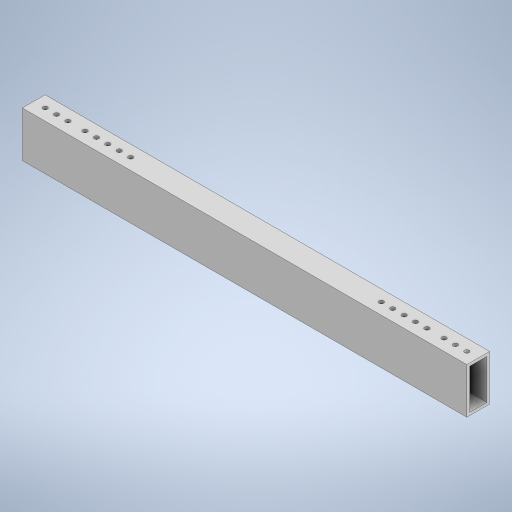
# Autodesk Inventor part: (a)swerveassembly
Saved by Autodesk Inventor 2024 (Build 280153000, 153)
## iProperties
Created: 2023-09-27
Part Number: (a)swerveassembly
Material: Generic
Document SubType Name: Modeling
Designer: s137416
Density: 1 g/cm^3
Appearance: Default
Author: s137416
Autodesk Inventor part; units mm, degrees
ref_plane "YZ Plane" through (0, 0, 0) normal (1, 0, 0) x (0, 1, 0)
ref_plane "XZ Plane" through (0, 0, 0) normal (0, 1, 0) x (-1, 0, 0)
ref_plane "XY Plane" through (0, 0, 0) normal (0, 0, 1) x (1, 0, 0)
sketch "Sketch1" plane through (0, 0, 0) normal (0, 0, 1) x (1, 0, 0)
  line L0 (-7.3593, 50.2532) -> (487.9407, 50.2532)
  line L1 (487.9407, 50.2532) -> (487.9407, -0.5468)
  line L2 (487.9407, -0.5468) -> (-7.3593, -0.5468)
  line L3 (-7.3593, -0.5468) -> (-7.3593, 50.2532)
  point P0 (0, 0)
  dimension "d0" = 495.3
  dimension "d1" = 50.8
  constraints: 8 end point, 2 parallel, 1 horizontal, 1 perpendicular
  measures "d0" distance of L1.end L2.end
  measures "d1" distance of L2.end L0.start
extrude "Extrusion1" add sketch "Sketch1" along normal blind 25.4
sketch "Sketch2" plane through (-7.3593, 50.2532, 0) normal (0, 1, 0) x (1, 0, 0)
  circle A0 centre (57.15, -12.7) radius 2.5019
  line L0 (0, 0) -> (0, -25.4) projected
  circle A1 centre (69.85, -12.7) radius 2.5019
  circle A2 centre (82.55, -12.7) radius 2.5019
  circle A3 centre (95.25, -12.7) radius 2.5019
  circle A4 centre (107.95, -12.7) radius 2.5019
  circle A5 centre (438.15, -12.7) radius 2.5019
  line L1 (495.3, 0) -> (495.3, -25.4) projected
  circle A6 centre (425.45, -12.7) radius 2.5019
  circle A7 centre (412.75, -12.7) radius 2.5019
  circle A8 centre (400.05, -12.7) radius 2.5019
  circle A9 centre (387.35, -12.7) radius 2.5019
  circle A10 centre (482.6, -12.7) radius 2.5019
  circle A11 centre (469.9, -12.7) radius 2.5019
  circle A12 centre (457.2, -12.7) radius 2.5019
  circle A13 centre (12.7, -12.7) radius 2.5019
  circle A14 centre (25.4, -12.7) radius 2.5019
  circle A15 centre (38.1, -12.7) radius 2.5019
  point P0 (7.3593, 0)
  dimension "d4" = 5.0038
  dimension "d5" = 57.15
  dimension "d6" = 5.0038
  dimension "d7" = 12.7
  dimension "d8" = 5.0038
  dimension "d9" = 5.0038
  dimension "d10" = 5.0038
  dimension "d11" = 12.7
  dimension "d12" = 12.7
  dimension "d13" = 12.7
  dimension "d14" = 5.0038
  dimension "d15" = 57.15
  dimension "d16" = 5.0038
  dimension "d17" = 12.7
  dimension "d18" = 5.0038
  dimension "d19" = 12.7
  dimension "d20" = 5.0038
  dimension "d21" = 12.7
  dimension "d22" = 5.0038
  dimension "d23" = 12.7
  dimension "d26" = 5.0038
  dimension "d27" = 5.0038
  dimension "d28" = 5.0038
  dimension "d29" = 12.7
  dimension "d30" = 12.7
  dimension "d31" = 12.7
  dimension "d32" = 5.0038
  dimension "d33" = 5.0038
  dimension "d34" = 5.0038
  dimension "d35" = 12.7
  dimension "d36" = 12.7
  dimension "d37" = 12.7
  constraints: 16 centre point
  measures "d4" diameter of A0
  measures "d5" distance from line of L0 A0.centre
  measures "d6" diameter of A1
  measures "d7" distance of A1.centre A0.centre
  measures "d8" diameter of A2
  measures "d9" diameter of A3
  measures "d10" diameter of A4
  measures "d11" distance of A1.centre A2.centre
  measures "d12" distance of A2.centre A3.centre
  measures "d13" distance of A3.centre A4.centre
  measures "d14" diameter of A5
  measures "d15" distance from line of L1 A5.centre
  measures "d16" diameter of A6
  measures "d17" distance of A5.centre A6.centre
  measures "d18" diameter of A7
  measures "d19" distance of A7.centre A6.centre
  measures "d20" diameter of A8
  measures "d21" distance of A7.centre A8.centre
  measures "d22" diameter of A9
  measures "d23" distance of A8.centre A9.centre
  measures "d26" diameter of A10
  measures "d27" diameter of A11
  measures "d28" diameter of A12
  measures "d29" distance from line of L1 A10.centre
  measures "d30" distance of A10.centre A11.centre
  measures "d31" distance of A11.centre A12.centre
  measures "d32" diameter of A13
  measures "d33" diameter of A14
  measures "d34" diameter of A15
  measures "d35" distance from line of L0 A13.centre
  measures "d36" distance of A13.centre A14.centre
  measures "d37" distance of A14.centre A15.centre
extrude "Extrusion2" cut sketch "Sketch2" against normal blind 50.8
shell "Shell1" thickness 3.175 removed faces 18 at (487.9407, 16.3866, 16.9333) at (475.14, 16.3866, 10.2001) at (462.44, 16.3866, 10.2001) at (449.74, 16.3866, 10.2001) at (432.7909, 16.3866, 11.197) at (417.99, 16.3866, 10.2001) at (405.29, 16.3866, 10.2001) at (20.5345, 16.3866, 12.9013) at (103.0845, 16.3866, 12.9013) at (392.59, 16.3866, 10.2001) at (-7.3593, 33.3199, 16.9333) at (7.8345, 16.3866, 12.9013) at (52.2845, 16.3866, 12.9013) at (33.2345, 16.3866, 12.9013) at (90.3845, 16.3866, 12.9013) at (64.9845, 16.3866, 12.9013) at (77.6845, 16.3866, 12.9013) at (379.89, 16.3866, 10.2001)
body "Solid1"
